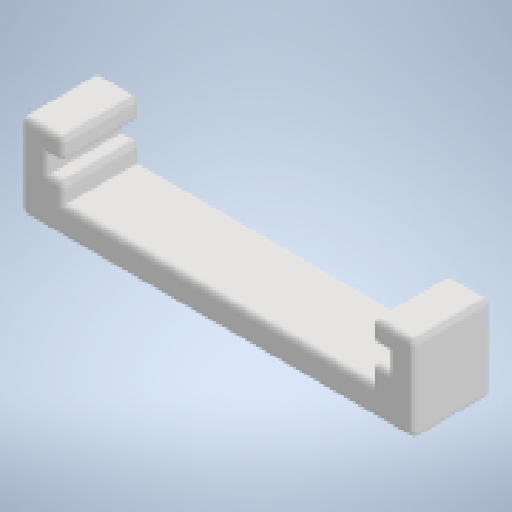
# Autodesk Inventor part: uMule-battery_cover
Saved by Autodesk Inventor 2024.2 (Build 282272000, 272)
## iProperties
Created: 2024-10-27
Part Number: uMule-battery_cover
Material: Ogólny
Document SubType Name: Modeling
Designer: owozn
Density: 1 g/cm^3
Appearance: Domyślna
Author: owozn
Autodesk Inventor part; units mm, degrees
ref_plane "YZ Plane" through (0, 0, 0) normal (1, 0, 0) x (0, 1, 0)
ref_plane "XZ Plane" through (0, 0, 0) normal (0, 1, 0) x (-1, 0, 0)
ref_plane "XY Plane" through (0, 0, 0) normal (0, 0, 1) x (1, 0, 0)
sketch "Szkic1" plane through (0, 0, 0) normal (0, 0, 1) x (1, 0, 0)
  line L0 (0, 0) -> (107, 0)
  line L1 (107, 0) -> (107, -5)
  line L2 (107, -5) -> (0, -5)
  line L3 (0, -5) -> (0, 0)
  line L4 (0, 0) -> (-6, 0)
  line L5 (-6, 0) -> (-6, -6)
  line L6 (-6, -6) -> (0, -6)
  line L7 (0, -6) -> (0, 0)
  line L8 (107, 0) -> (113, 0)
  line L9 (113, 0) -> (113, -6)
  line L10 (113, -6) -> (107, -6)
  line L11 (107, -6) -> (107, 0)
  line L12 (122.5, 7.5) -> (107.5, 7.5)
  line L13 (107.5, 7.5) -> (107.5, -12.5)
  line L14 (107.5, -12.5) -> (122.5, -12.5)
  line L15 (122.5, -12.5) -> (122.5, 7.5)
  line L16 (122.5, 7.5) -> (107.5, -12.5) construction
  line L17 (107.5, 7.5) -> (122.5, -12.5) construction
  line L18 (53.5, 0) -> (53.5, -20) construction
  line L19 (-15.5, 7.5) -> (-0.5, 7.5)
  line L20 (-0.5, 7.5) -> (-0.5, -12.5)
  line L21 (-0.5, -12.5) -> (-15.5, -12.5)
  line L22 (-15.5, -12.5) -> (-15.5, 7.5)
  line L23 (-15.5, -12.5) -> (122.5, -12.5)
  line L24 (122.5, -12.5) -> (122.5, -22.5)
  line L25 (122.5, -22.5) -> (-15.5, -22.5)
  line L26 (-15.5, -22.5) -> (-15.5, -12.5)
  point P0 (115, -2.5)
  point P1 (107.5, -6)
  point P2 (107.5, 0)
  point P3 (-0.5, 0)
  point P4 (-0.5, -6)
  dimension "d0" = 107
  dimension "d1" = 5
  dimension "d2" = 6
  dimension "d3" = 6
  dimension "d4" = 6
  dimension "d5" = 15
  dimension "d6" = 20
  dimension "d7" = 0.5
  dimension "d8" = 2.5
  dimension "d9" = 20
  dimension "d12" = 10
  dimension "d13" = 138
  constraints: 54 end point, 10 parallel, 5 horizontal, 5 perpendicular, 4 symmetric about line, 3 midpoint, 1 point on line, 1 vertical
  measures "d0" distance of L1.end L2.end
  measures "d1" distance of L0.end L1.end
  measures "d2" distance of L6.end L5.end
  measures "d3" distance of L5.end L4.end
  measures "d4" distance of L9.end L10.end
  measures "d5" distance of L14.end L13.end
  measures "d6" distance of L13.end L12.end
  measures "d7" distance between parallel lines of L1 L13
  measures "d8" vertical distance of L0.start point (115, -2.5)
  measures "d9" distance of L18.start L18.end
  measures "d12" distance of L23.end L24.end
  measures "d13" distance of L24.end L25.end
extrude "Wyciągnięcie proste1" add sketch "Szkic1" along normal blind 27 contours L4 L5 L6 L20 L21 L22 L19 | L13 L12 L15 L14 L10 L9 L8 | L23 L14 L24 L25 L26 L21
fillet "Zaokrąglenie1" radius 2 42 edges at (107.5, -9.25, 0) (110.25, -6, 0) (113, -3, 0) (110.25, 0, 0) (107.5, 3.75, 0) (110.25, 0, 27) (107.5, 3.75, 27) (113, -3, 27) (110.25, -6, 27) (107.5, -9.25, 27) (53.5, -12.5, 27) (-0.5, -9.25, 27) (-6, -3, 27) (-3.25, 0, 27) (-3.25, -6, 27) (-0.5, 3.75, 27) (-0.5, 0, 13.5) (107.5, 0, 13.5) (-0.5, 3.75, 0) (-3.25, 0, 0) (-6, -3, 0) (-3.25, -6, 0) (-0.5, -9.25, 0) (53.5, -12.5, 0) (-8, 7.5, 0) (-15.5, -7.5, 0) (53.5, -22.5, 0) (122.5, -7.5, 0) (115, 7.5, 0) (122.5, 7.5, 13.5) (122.5, -7.5, 27) (122.5, -22.5, 13.5) (53.5, -22.5, 27) (115, 7.5, 27) (-8, 7.5, 27) (-15.5, -7.5, 27) (-0.5, 7.5, 13.5) (107.5, 7.5, 13.5) (107.5, -6, 13.5) (-0.5, -6, 13.5) (-15.5, 7.5, 13.5) (-15.5, -22.5, 13.5)
